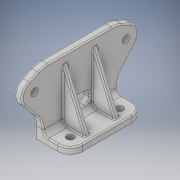
# Autodesk Inventor part: SharpIRsensorMount
Saved by Autodesk Inventor 2017 (Build 210142000, 142)
## iProperties
Created: 2017-09-15
Part Number: SharpIRsensorMount
Material: Generic
Document SubType Name: Modeling
Designer: Axel
Density: 1 g/cm^3
Appearance: Default
Author: Axel
Autodesk Inventor part; units mm, degrees
ref_plane "YZ Plane" through (0, 0, 0) normal (1, 0, 0) x (0, 1, 0)
ref_plane "XZ Plane" through (0, 0, 0) normal (0, 1, 0) x (-1, 0, 0)
ref_plane "XY Plane" through (0, 0, 0) normal (0, 0, 1) x (1, 0, 0)
sketch "Sketch1" plane through (0, 0, 0) normal (0, 1, 0) x (-1, 0, 0)
  circle A0 centre (0, 10) radius 1.5
  arc A1 (0, 15) -> (-5, 10) centre (0, 10) ccw
  circle A2 centre (0, -10) radius 1.5
  arc A3 (-5, -10) -> (0, -15) centre (0, -10) ccw
  line L0 (-5, 10) -> (-5, -10)
  line L1 (0, 15) -> (9, 15)
  line L2 (9, 15) -> (9, -15)
  line L3 (9, -15) -> (0, -15)
  point P0 (0, 0)
  point P1 (-5, 0)
  dimension "d0" = 3
  dimension "d1" = 10
  dimension "d2" = 3
  dimension "d3" = 10
  dimension "d4" = 20
  dimension "d6" = 14
  dimension "d7" = 30
  constraints: 8 end point, 4 centre point, 4 point on circle, 2 coincident, 2 tangent, 2 vertical alignment, 1 horizontal alignment, 1 midpoint, 1 parallel, 1 perpendicular, 1 vertical
  measures "d0" diameter of A0
  measures "d1" diameter of A1
  measures "d2" diameter of A2
  measures "d3" diameter of A3
  measures "d4" distance of A2.centre A0.centre
  measures "d6" distance between parallel lines of L0 L2
  measures "d7" distance between parallel lines of L3 L1
extrude "Extrusion1" add sketch "Sketch1" along normal blind 3
sketch "Sketch2" plane through (-9, 0, -15) normal (-1, 0, 0) x (0, 0, 1)
  circle A0 centre (-3.5, 20) radius 1.5
  circle A1 centre (33.5, 20) radius 1.5
  arc A2 (-5.5119, 24.5774) -> (-7.3393, 16.7969) centre (-3.5, 20) ccw
  arc A3 (37.3393, 16.7969) -> (35.5119, 24.5774) centre (33.5, 20) ccw
  line L0 (30, 0) -> (0, 0) projected
  line L1 (0, 3) -> (30, 3) projected
  line L2 (0, 0) -> (0, 3) projected
  line L3 (30, 3) -> (0, 3)
  line L4 (0, 3) -> (0, 5.101)
  line L5 (-1.8572, 10.226) -> (-7.3393, 16.7969)
  line L6 (30, 3) -> (30, 5.101)
  line L7 (31.8572, 10.226) -> (37.3393, 16.7969)
  arc A4 (0, 5.101) -> (-1.8572, 10.226) centre (-8, 5.101) ccw
  arc A5 (31.8572, 10.226) -> (30, 5.101) centre (38, 5.101) ccw
  line L8 (11, 10) -> (19, 10)
  line L9 (19, 10) -> (19, 5)
  line L10 (19, 5) -> (11, 5)
  line L11 (11, 5) -> (11, 10)
  line L12 (30, 27) -> (0, 27)
  line L13 (0, 27) -> (-5.5119, 24.5774)
  line L14 (30, 27) -> (35.5119, 24.5774)
  point P0 (15, 0)
  point P1 (15, 25)
  point P2 (15, 0)
  point P3 (0, 8)
  point P4 (30, 8)
  point P5 (15, 0)
  point P6 (15, 5)
  point P7 (15, 0)
  dimension "d10" = 3
  dimension "d11" = 3
  dimension "d12" = 10
  dimension "d13" = 10
  dimension "d14" = 37
  dimension "d15" = 20
  dimension "d16" = 5
  dimension "d17" = 5
  dimension "d18" = 8
  dimension "d22" = 8
  dimension "d23" = 5
  dimension "d24" = 2
  dimension "d40" = 15
  dimension "d41" = 15
  constraints: 24 end point, 8 point on circle, 8 tangent, 6 centre point, 4 midpoint, 4 point on line, 2 coincident, 2 horizontal, 2 parallel, 2 perpendicular, 2 vertical alignment, 1 equal radius, 1 horizontal alignment, 1 vertical
  measures "d10" diameter of A0
  measures "d11" diameter of A1
  measures "d12" diameter of A2
  measures "d13" diameter of A3
  measures "d14" distance of A1.centre A0.centre
  measures "d15" distance from line of A1.centre L0
  measures "d16" distance of L1.start point (0, 8)
  measures "d17" distance of L1.end point (30, 8)
  measures "d18" radius of A4
  measures "d22" distance of L9.end L10.end
  measures "d23" distance of L8.end L9.end
  measures "d24" distance between parallel lines of L10 L1
  measures "d40" horizontal distance of point (15, 25) L12.start
  measures "d41" horizontal distance of point (15, 25) L12.end
extrude "Extrusion2" add sketch "Sketch2" against normal blind 3
fillet "Fillet1" radius 2 5 edges at (-6, 3, 0) (-7.5, 5, -4) (-7.5, 10, -4) (-7.5, 5, 4) (-7.5, 10, 4)
sketch "Sketch3" plane through (-6, 0, -15) normal (1, 0, 0) x (0, 0, -1)
  line L0 (-20, 0) -> (-22, 0)
  line L1 (-22, 0) -> (-22, 24)
  line L2 (-22, 24) -> (-20, 24)
  line L3 (-20, 24) -> (-20, 0)
  line L4 (-30, 0.5) -> (-30, 5.101) projected
  line L5 (-10, 24) -> (-8, 24)
  line L6 (-8, 24) -> (-8, 0)
  line L7 (-8, 0) -> (-10, 0)
  line L8 (-10, 0) -> (-10, 24)
  point P0 (-15, 0)
  point P1 (-25, 0)
  point P2 (0, 0.5)
  point P3 (-5, 0)
  dimension "d29" = 2
  dimension "d30" = 24
  dimension "d31" = 8
  dimension "d32" = 2
  dimension "d33" = 24
  dimension "d34" = 8
  constraints: 16 end point, 4 parallel, 2 horizontal, 2 horizontal alignment, 2 perpendicular
  measures "d29" distance of L1.end L2.end
  measures "d30" distance of L0.end L1.end
  measures "d31" distance between parallel lines of L4 L1
  measures "d32" distance of L6.end L7.end
  measures "d33" distance of L5.end L6.end
  measures "d34" distance from line of point (0, 0.5) L6
extrude "Extrusion3" add sketch "Sketch3" along normal blind 9
sketch "Sketch4" plane through (-6, 5, -7) normal (0, 0, -1) x (-1, 0, 0)
  line L0 (-9, -2) -> (-2, -2) projected
  line L1 (0, 19) -> (-9, 19) projected
  line L2 (-9, -2) -> (0, 19)
  line L3 (0, 19) -> (-14.4459, 19.4914)
  line L4 (-14.4459, 19.4914) -> (-9, -2)
  point P0 (-6, -5)
  constraints: 6 end point
extrude "Extrusion4" cut sketch "Sketch4" against normal blind 20
fillet "Fillet3" radius 0.5 20 edges at (-5.4142, 3.5858, -7) (-0.5001, 3, -7) (-6, 14.5, -7) (-5.4142, 3.5858, -5) (-0.5001, 3, -5) (-6, 14.5, -5) (-1.5, 13.5, -5) (-1.5, 13.5, -7) (-6, 24, -6) (3, 3, -6) (-1.5, 13.5, 7) (-6, 14.5, 7) (-5.4142, 3.5858, 7) (-0.5001, 3, 7) (-1.5, 13.5, 5) (-0.5001, 3, 5) (-5.4142, 3.5858, 5) (-6, 14.5, 5) (3, 3, 6) (-6, 24, 6)
fillet "Fillet4" radius 10 2 edges at (-7.5, 27, 15) (-7.5, 27, -15)
fillet "Fillet5" radius 0.5 55 edges at (-9, 7.8266, 15.4786) (-6, 7.8266, 15.4786) (-9, 13.5114, 19.5982) (-9, 21.1432, 23.3675) (-9, 25.3661, 18.7175) (-9, 26.7864, 14.9551) (-9, 27, 0) (-9, 26.7864, -14.9551) (-9, 25.3661, -18.7175) (-9, 21.1432, -23.3675) (-9, 13.5114, -19.5982) (-9, 7.8266, -15.4786) (-9, 2.5505, -15) (-9, 2.5505, 15) (-6, 5.0505, 15) (-5.4142, 3.5858, 15) (-2, 3, 15) (3.5355, 3, 13.5355) (5, 3, 0) (3.5355, 3, -13.5355) (-2.0001, 3, -15) (-5.4142, 3.5858, -15) (-6, 5.0505, -15) (-6, 7.8266, -15.4786) (-6, 13.5114, -19.5982) (-6, 21.1432, -23.3675) (-6, 25.3661, -18.7175) (-6, 26.7864, -14.9551) (-6, 27, 0) (-6, 26.7864, 14.9551) (-6, 25.3661, 18.7175) (-6, 21.1432, 23.3675) (-6, 13.5114, 19.5982) (-9, 10, 0) (-6, 10, 0) (-9, 9.4142, 3.4142) (-9, 7.5, 4) (-9, 5.5858, 3.4142) (-9, 5, 0) (-9, 5.5858, -3.4142) (-9, 7.5, -4) (-9, 9.4142, -3.4142) (-6, 9.4142, -3.4142) (-6, 7.5, -4) (-6, 5.5858, -3.4142) (-6, 5, 0) (-6, 5.5858, 3.4142) (-6, 7.5, 4) (-6, 9.4142, 3.4142) (-4.5, 0, -15) (3.5355, 0, -13.5355) (5, 0, 0) (3.5355, 0, 13.5355) (-4.5, 0, 15) (-9, 0, 0)
body "Solid1"
